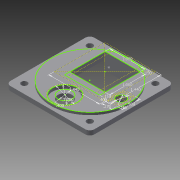
# Autodesk Inventor part: icarus-sam-instrument-mount
Saved by Autodesk Inventor 2015 (Build 190159000, 159)
## iProperties
Created: 2016-01-17
Part Number: icarus-sam-instrument-mount
Material: Generic
Document SubType Name: Modeling
Designer: bovine
Density: 1 g/cm^3
Appearance: Default
Author: bovine
Autodesk Inventor part; units mm, degrees
ref_plane "YZ Plane" through (0, 0, 0) normal (1, 0, 0) x (0, 1, 0)
ref_plane "XZ Plane" through (0, 0, 0) normal (0, 1, 0) x (-1, 0, 0)
ref_plane "XY Plane" through (0, 0, 0) normal (0, 0, 1) x (1, 0, 0)
sketch "Sketch1" plane through (0, 0, 0) normal (0, 1, 0) x (-1, 0, 0)
  line L0 (30.1625, 30.1625) -> (-30.1625, 30.1625)
  line L1 (-30.1625, 30.1625) -> (-30.1625, -30.1625)
  line L2 (-30.1625, -30.1625) -> (30.1625, -30.1625)
  line L3 (30.1625, -30.1625) -> (30.1625, 30.1625)
  circle A0 centre (0, 0) radius 33.3375 construction
  circle A1 centre (0, 0) radius 28.575
  line L4 (-30.1625, 30.1625) -> (30.1625, -30.1625) construction
  line L5 (30.1625, 30.1625) -> (-30.1625, -30.1625) construction
  circle A2 centre (23.5732, 23.5732) radius 2.159
  circle A3 centre (23.5732, -23.5732) radius 2.159
  circle A4 centre (-23.5732, 23.5732) radius 2.159
  circle A5 centre (-23.5732, -23.5732) radius 2.159
  point P0 (0, 0)
  point P1 (0, 0)
  dimension "d0" = 60.325
  dimension "d1" = 60.325
  dimension "d2" = 66.675
  dimension "d3" = 57.15
  dimension "d4" = 4.318
  dimension "d5" = 4.318
  dimension "d6" = 4.318
  dimension "d7" = 4.318
  constraints: 12 end point, 6 centre point, 4 point on circle, 4 point on line, 3 coincident, 2 parallel, 1 horizontal, 1 midpoint, 1 perpendicular
  measures "d0" distance of L2.end L1.end
  measures "d1" distance of L1.end L0.end
  measures "d2" diameter of A0
  measures "d3" diameter of A1
  measures "d4" diameter of A2
  measures "d5" diameter of A3
  measures "d6" diameter of A4
  measures "d7" diameter of A5
extrude "Extrusion1" add sketch "Sketch1" along normal blind 3.175 contours L3 L2 L1 L0 | A1
sketch "Sketch2" plane through (0, 3.175, 0) normal (0, 1, 0) x (1, 0, 0)
  circle A0 centre (0, 0) radius 27.94
  circle A1 centre (0, 0) radius 28.575 construction
  point P0 (0, 0)
  dimension "d10" = 55.88
  dimension "d17" = 57.15
  constraints: 2 centre point, 2 coincident
  measures "d10" diameter of A0
  measures "d17" diameter of A1
extrude "Extrusion2" add sketch "Sketch2" along normal blind 1.905
fillet "Fillet1" radius 3.175 4 edges at (30.1625, 1.5875, 30.1625) (-30.1625, 1.5875, 30.1625) (30.1625, 1.5875, -30.1625) (-30.1625, 1.5875, -30.1625)
sketch "Sketch3" plane through (0, 5.08, 0) normal (0, 1, 0) x (1, 0, 0)
  line L0 (-12.7, -1.8506) -> (12.7, -1.8506)
  line L1 (12.7, -1.8506) -> (12.7, 23.5494)
  line L2 (12.7, 23.5494) -> (-12.7, 23.5494)
  line L3 (-12.7, 23.5494) -> (-12.7, -1.8506)
  circle A0 centre (0, 0) radius 27.94
  circle A1 centre (0, 0) radius 27.94 construction
  circle A2 centre (0.0007, -17.939) radius 5.08
  line L4 (16.9084, 0) -> (27.94, 0) construction
  circle A3 centre (22.4242, 0) radius 3.302
  circle A4 centre (0.0007, -17.939) radius 9.017
  line L5 (-12.7, 23.5494) -> (12.7, 23.5494)
  line L6 (12.7, 23.5494) -> (12.7, 27.3594)
  line L7 (12.7, 27.3594) -> (-12.7, 27.3594)
  line L8 (-12.7, 27.3594) -> (-12.7, 23.5494)
  line L9 (-12.7, -1.8506) -> (12.7, -1.8506)
  line L10 (12.7, -1.8506) -> (12.7, -5.6606)
  line L11 (12.7, -5.6606) -> (-12.7, -5.6606)
  line L12 (-12.7, -5.6606) -> (-12.7, -1.8506)
  circle A5 centre (0, 0) radius 27.94 construction
  line L13 (9.7799, 26.1725) -> (9.7799, -5.6606) construction
  line L14 (-10.16, 27.3594) -> (-10.16, -5.6606) construction
  circle A6 centre (22.4242, 0) radius 5.08 construction
  line L15 (-18.288, 29.1374) -> (18.288, 29.1374) construction
  line L16 (18.288, 29.1374) -> (18.288, -7.4386) construction
  line L17 (18.288, -7.4386) -> (-18.288, -7.4386) construction
  line L18 (-18.288, -7.4386) -> (-18.288, 29.1374) construction
  line L19 (-18.288, 29.1374) -> (18.288, -7.4386) construction
  line L20 (18.288, 29.1374) -> (-18.288, -7.4386) construction
  line L21 (18.9952, 6.35) -> (25.8532, 6.35) construction
  line L22 (25.8532, 6.35) -> (25.8532, -6.35) construction
  line L23 (25.8532, -6.35) -> (18.9952, -6.35) construction
  line L24 (18.9952, -6.35) -> (18.9952, 6.35) construction
  line L25 (18.9952, 6.35) -> (25.8532, -6.35) construction
  line L26 (25.8532, 6.35) -> (18.9952, -6.35) construction
  circle A7 centre (0.0007, -17.939) radius 9.525 construction
  point P0 (0, 10.8494)
  dimension "d18" = 25.4
  dimension "d19" = 25.4
  dimension "d32" = 10.16
  dimension "d33" = 6.604
  dimension "d34" = 18.034
  dimension "d37" = 3.81
  dimension "d38" = 3.81
  dimension "d48" = 10.16
  dimension "d49" = 36.576
  dimension "d50" = 36.576
  dimension "d51" = 6.858
  dimension "d52" = 12.7
  dimension "d53" = 19.05
  constraints: 54 end point, 10 parallel, 7 perpendicular, 5 centre point, 5 horizontal, 5 midpoint, 4 point on line, 3 coincident, 2 horizontal alignment, 5 other
  measures "d18" distance of L2.end L1.end
  measures "d19" distance of L1.end L0.end
  measures "d32" diameter of A2
  measures "d33" diameter of A3
  measures "d34" diameter of A4
  measures "d37" distance of L6.end L5.end
  measures "d38" distance of L9.end L10.end
  measures "d48" diameter of A6
  measures "d49" distance of L16.end L17.end
  measures "d50" distance of L15.end L16.end
  measures "d51" distance of L22.end L23.end
  measures "d52" distance of L21.end L22.end
  measures "d53" diameter of A7
extrude "Extrusion4" cut sketch "Sketch3" against normal through all contours L3 L2 L1 L0 | A2 | A3
extrude "Extrusion5" cut sketch "Sketch3" against normal blind 2.54 contours A4
extrude "Extrusion6" add sketch "Sketch3" against normal blind 11.811 separate body contours L0 L10 L11 L12 | L8 A0 L7 L6 L2 | L8 L7 A0 | A0 L7 L6
sketch "Sketch4" plane through (-12.7, 5.08, 5.6606) normal (0, 0, 1) x (1, 0, 0)
  line L0 (25.4, -8.255) -> (0, -8.255) construction
  line L1 (25.4, 0) -> (25.4, -11.811) construction
  line L2 (0, 0) -> (0, -11.811) construction
  point P0 (12.7, -5.08)
  point P1 (2.5418, -8.255)
  point P2 (22.8582, -8.255)
  constraints: 4 point on line, 2 end point, 1 horizontal
hole "Hole1" at (10.1582, -3.175, 5.6606) at (-10.1582, -3.175, 5.6606) direction (0, 0, -1) diameter 2.032 end through all bodies 2
combine bodies "Combine1" operation type add bodies to combine 1 2
delete faces "Delete1" heal yes whole lump no faces at (10.3555, 4.445, -27.3594) (-8.0109, 4.445, -27.3594) (12.7, 3.81, -26.5352) (-12.7, 3.81, -25.711)
body "Solid2"
